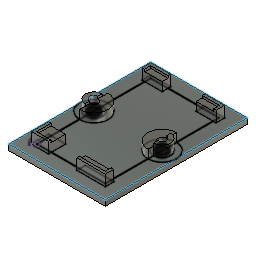
bldc_pcb_v4_holder (Autodesk Fusion 360 design; units mm, degrees)
Autodesk Fusion 360 part; units mm, degrees
note: some values were not read from the file. Chosen so that the rebuilt part matches the saved one: which bodies a step acts on. Set by a fixed rule: which sketch regions a step uses.
sketch "Sketch1" plane through (0, 0, 0) normal (0, 0, 1) x (1, 0, 0)
  line L0 (0, 0) -> (24, 0)
  line L1 (24, 0) -> (24, 40)
  line L2 (24, 40) -> (0, 40)
  line L3 (0, 40) -> (0, 0)
  circle A0 centre (0, 20) radius 5
  circle A1 centre (24, 20) radius 5
  circle A2 centre (0, 20) radius 1.5
  circle A3 centre (0, 20) radius 3
  circle A4 centre (24, 20) radius 1.5
  circle A5 centre (24, 20) radius 3
  line L4 (0, 38) -> (6, 38)
  line L5 (6, 38) -> (6, 40)
  line L6 (24, 38) -> (18, 38)
  line L7 (18, 38) -> (18, 40)
  line L8 (24, 2) -> (15, 2)
  line L9 (15, 2) -> (15, 0)
  line L10 (0, 0) -> (5, 0)
  line L11 (5, 0) -> (5, 5)
  line L12 (5, 5) -> (0, 5)
  line L13 (0, 5) -> (0, 0)
  line L14 (-5, -5) -> (29, -5)
  line L15 (29, -5) -> (29, 45)
  line L16 (29, 45) -> (-5, 45)
  line L17 (-5, 45) -> (-5, -5)
  circle A6 centre (24, 20) radius 2
  circle A7 centre (0, 20) radius 2
  line L18 (-0.1, -0.1) -> (24.1, -0.1)
  line L19 (24.1, -0.1) -> (24.1, 40.1)
  line L20 (24.1, 40.1) -> (-0.1, 40.1)
  line L21 (-0.1, 40.1) -> (-0.1, -0.1)
  line L22 (6, 40) -> (6, 41)
  line L23 (0, 38) -> (-1, 38)
  line L24 (-1, 38) -> (-1, 41)
  line L25 (-1, 41) -> (6, 41)
  line L26 (18, 40) -> (18, 41)
  line L27 (24, 38) -> (25, 38)
  line L28 (25, 38) -> (25, 41)
  line L29 (25, 41) -> (18, 41)
  line L30 (24, 2) -> (25, 2)
  line L31 (15, 0) -> (15, -1)
  line L32 (25, 2) -> (25, -1)
  line L33 (25, -1) -> (15, -1)
  line L34 (0, 5) -> (-1, 5)
  line L35 (5, 0) -> (5, -1)
  line L36 (-1, 5) -> (-1, -1)
  line L37 (-1, -1) -> (5, -1)
  dimension "d1" = 24
  dimension "d2" = 40
  dimension "d3" = 10
  dimension "d4" = 10
  dimension "d5" = 3
  dimension "d6" = 6
  dimension "d7" = 3
  dimension "d8" = 6
  dimension "d9" = 6
  dimension "d10" = 2
  dimension "d11" = 6
  dimension "d12" = 2
  dimension "d13" = 9
  dimension "d14" = 2
  dimension "d15" = 5
  dimension "d16" = 5
  dimension "d27" = 4
  dimension "d28" = 4
  dimension "d29" = 0.1
  dimension "d30" = 0.1
  dimension "d31" = 0.1
  dimension "d32" = 0.1
  dimension "d33" = 1
  dimension "d34" = 1
  dimension "d35" = 1
  dimension "d36" = 1
  dimension "d37" = 1
  dimension "d38" = 1
  dimension "d39" = 1
  dimension "d40" = 1
  constraint horizontal L0
  constraint vertical L1
  constraint horizontal L2
  constraint vertical L3
  constraint coincident L0.start L3.end
  constraint midpoint L3 A0.centre
  constraint midpoint L1 A1.centre
  constraint concentric A0 A2
  constraint concentric A0 A3
  constraint concentric A1 A4
  constraint concentric A1 A5
  constraint coincident L3 L4.start
  constraint perpendicular L3 L4
  constraint coincident L2 L5.end
  constraint perpendicular L2 L5
  constraint coincident L1 L6.start
  constraint perpendicular L1 L6
  constraint coincident L2 L7.end
  constraint perpendicular L2 L7
  constraint coincident L1 L8.start
  constraint perpendicular L1 L8
  constraint coincident L0 L9.end
  constraint perpendicular L0 L9
  constraint horizontal L10
  constraint vertical L11
  constraint horizontal L12
  constraint vertical L13
  constraint horizontal L14
  constraint vertical L15
  constraint horizontal L16
  constraint vertical L17
  constraint concentric A1 A6
  constraint concentric A0 A7
  constraint horizontal L18
  constraint vertical L19
  constraint horizontal L20
  constraint vertical L21
  constraint perpendicular L2 L22
  constraint perpendicular L3 L23
  constraint perpendicular L23 L24
  constraint perpendicular L22 L25
  constraint perpendicular L2 L26
  constraint perpendicular L19 L27
  constraint perpendicular L27 L28
  constraint perpendicular L26 L29
  constraint perpendicular L19 L30
  constraint perpendicular L18 L31
  constraint perpendicular L18 L32
  constraint perpendicular L31 L33
  constraint perpendicular L13 L34
  constraint perpendicular L10 L35
  constraint perpendicular L34 L36
  constraint perpendicular L35 L37
  measures "d1" distance of L0.start L0.end
  measures "d2" distance of L0.start L2.end
  measures "d3" diameter of A0
  measures "d4" diameter of A1
  measures "d5" diameter of A2
  measures "d6" diameter of A3
  measures "d7" diameter of A4
  measures "d8" diameter of A5
  measures "d9" distance of L4.start L4.end
  measures "d10" distance of L4.end L5.end
  measures "d11" distance of L6.start L6.end
  measures "d12" distance of L6.end L7.end
  measures "d13" distance of L8.start L8.end
  measures "d14" distance of L8.end L9.end
  measures "d15" distance of L0.start L10.end
  measures "d16" distance of L0.start L12.end
  measures "d27" diameter of A6
  measures "d28" diameter of A7
  measures "d29" distance of L1 L19
  measures "d30" distance of L3 L21
  measures "d31" distance of L2 L20
  measures "d32" distance of L0 L18
  measures "d33" distance of L5.end L22.end
  measures "d34" distance of L4.start L23.end
  measures "d35" distance of L7.end L26.end
  measures "d36" distance of L6.start L27.end
  measures "d37" distance of L8.start L30.end
  measures "d38" distance of L9.end L31.end
  measures "d39" distance of L12.end L34.end
  measures "d40" distance of L10.end L35.end
extrude "Extrude1" add sketch "Sketch1" along normal blind 3 contours L0 L3 L10 L11 L12 L13 | L0 L3 L10 L13 L18 L21 L34 L35 | L0 L1 L8 L9 | L0 L1 L18 L19 L30 L31 | L3 A0 A3 L21 | L3 A0 A3 | L3 A3 A7 L21 | L3 A3 A7 | L3 A2 A7 L21 | L3 A2 A7 | L3 A0 A3 L21 | L1 A1 A5 | L1 A1 A5 L19 | L3 A3 A7 L21 | L2 L3 L20 L21 L22 L23 | L2 L3 L4 L5 | L1 A5 A6 | L1 A5 A6 L19 | L1 A1 A5 L19 | L3 A2 A7 L21 | L1 A4 A6 | L1 A4 A6 L19 | L1 A5 A6 L19 | L1 L2 L6 L7 | L1 L2 L19 L20 L26 L27 | L1 A4 A6 L19 makes body 1 at (3.9667, 40.1, 1) makes body 2 at (22.0667, 40.1, 1) makes body 3 at (1.6, 3.3, 0) makes body 4 at (18.0333, 2, 1) makes body 5 at (0.3817, 15.0146, 2) makes body 6 at (19.0232, 19.5187, 1)
extrude "Extrude2" add sketch "Sketch1" along normal blind 3.8 contours L18 L21 L34 L35 L36 L37 | L18 L19 L30 L31 L32 L33 | A3 A7 L21 | A2 A7 L21 | L1 A5 A6 L19 | L20 L21 L22 L23 L24 L25 | L1 A4 A6 L19 | L1 A5 A6 L19 | A5 A6 L19 | L1 A4 A6 L19 | A4 A6 L19 | L19 L20 L26 L27 L28 L29 bodies 6 1 5 4 2 3
extrude "Extrude7" add sketch "Sketch1" against normal blind 2 bodies 1 6 5 4 2 3
extrude "Extrude8" cut sketch "Sketch1" along normal blind 1 and the other way blind 2 contours L3 A2 A7 L21 | L3 A2 A7 | L3 A2 L21 | L3 A2 | A2 A7 L21 | L3 A2 A7 L21 | A2 L21 | L1 A4 A6 | L1 A4 A6 L19 | L1 A4 | L1 A4 L19 | L1 A4 A6 L19 | A4 A6 L19 | A4 L19 bodies 1
